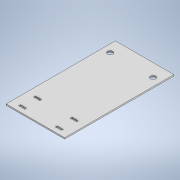
# Autodesk Inventor part: Platte1_2
Saved by Autodesk Inventor 2022 (Build 260153000, 153)
## iProperties
Created: 2022-04-02
Part Number: Platte1_2
Material: Generic
Document SubType Name: Modeling
Designer: benni
Density: 1 g/cm^3
Appearance: Default
Author: benni
Autodesk Inventor part; units mm, degrees
ref_plane "YZ Plane" through (0, 0, 0) normal (1, 0, 0) x (0, 1, 0)
ref_plane "XZ Plane" through (0, 0, 0) normal (0, 1, 0) x (-1, 0, 0)
ref_plane "XY Plane" through (0, 0, 0) normal (0, 0, 1) x (1, 0, 0)
sketch "Sketch1" plane through (0, 0, 0) normal (0, 1, 0) x (-1, 0, 0)
  line L0 (0, 0) -> (45, 0)
  line L1 (45, 0) -> (45, -84)
  line L2 (45, -84) -> (0, -84)
  line L3 (0, -84) -> (0, 0)
  line L4 (0, 0) -> (45, 0)
  line L5 (0, 2) -> (0, 0)
  circle A0 centre (6, -74) radius 2
  circle A1 centre (39, -74) radius 2
  line L6 (22.5, 0) -> (22.5, -84)
  line L7 (45, -10) -> (0, -10)
  line L8 (6, -3.5) -> (10.7625, -3.5)
  line L9 (10.7625, -3.5) -> (10.7625, -5)
  line L10 (10.7625, -5) -> (6, -5)
  line L11 (6, -5) -> (6, -3.5)
  line L12 (6, -16.5) -> (10.7625, -16.5)
  line L13 (10.7625, -16.5) -> (10.7625, -15)
  line L14 (10.7625, -15) -> (6, -15)
  line L15 (6, -15) -> (6, -16.5)
  line L16 (39, -3.5) -> (34.2375, -3.5)
  line L17 (34.2375, -3.5) -> (34.2375, -5)
  line L18 (34.2375, -5) -> (39, -5)
  line L19 (39, -5) -> (39, -3.5)
  line L20 (34.2375, -16.5) -> (34.2375, -15)
  line L21 (39, -15) -> (39, -16.5)
  line L22 (39, -16.5) -> (34.2375, -16.5)
  line L23 (34.2375, -15) -> (39, -15)
  dimension "d0" = 45
  dimension "d1" = 84
  dimension "d3" = 10
  dimension "d4" = 6
  dimension "d5" = 10
  dimension "d6" = 6
  dimension "d7" = 4
  dimension "d8" = 4
  dimension "d19" = 20
  dimension "d20" = 6
  dimension "d21" = 10
  dimension "d22" = 1.5
  constraints: 48 end point, 12 symmetric about line, 4 parallel, 3 horizontal, 3 perpendicular, 2 centre point, 2 coincident, 2 midpoint, 2 point on line
  measures "d0" distance of L1.end L2.end
  measures "d1" distance of L0.end L1.end
  measures "d3" distance from line of L2 point (6, -74)
  measures "d4" distance from line of L3 point (6, -74)
  measures "d5" distance from line of L2 point (39, -74)
  measures "d6" distance from line of L1 point (39, -74)
  measures "d7" diameter of A0
  measures "d8" diameter of A1
  measures "d19" diameter of L0 L7
  measures "d20" distance between parallel lines of L11 L3
  measures "d21" diameter of L10 L7
  measures "d22" distance of L8.end L9.end
extrude "Extrusion4" add sketch "Sketch1" along normal blind 1
body "Solid3"
